Autodesk Fusion 360 part; units mm, degrees
(part 2 of 2)
  constraint coincident L500 L639.end
  constraint perpendicular L500 L639
  constraint coincident L499 L640.start
  constraint coincident L501 L640.end
  constraint perpendicular L501 L640
  constraint coincident L500 L641.end
  constraint perpendicular L500 L641
  constraint coincident L495 L642.end
  constraint perpendicular L495 L642
  constraint coincident L495 L643.end
  constraint perpendicular L495 L643
  constraint coincident L495 L644.start
  constraint coincident L496 L644.end
  constraint perpendicular L496 L644
  measures "d1" distance of L345 L502
  measures "d2" distance of L432 L500
  measures "d3" distance of L12 L501
  measures "d4" distance of L477 L499
  measures "d5" distance of L243 L498
  measures "d6" distance of L284 L497
  measures "d7" distance of L115 L496
  measures "d8" distance of L74 L495
  measures "d9" distance of L196 L494
  measures "d10" distance of L208 L493
extrude "Extrude1" add sketch "b27d7a26cd9df215f168af8e672502c9323f781d_switch" against normal blind 3 contours L51 L301 L303 L501 L579 | L40 L62 L499 L501 L580 L581 | L303 L500 L501 L630 | L301 L492 L499 L579 | L492 L498 L499 L635 | L303 L387 L500 L502 L620 | L32 L429 L499 L501 L582 L583 | L325 L492 L498 L635 | L303 L304 L320 L502 | L305 L325 L497 L635 | L373 L382 L500 L502 L618 L619 | L291 L302 L328 L498 L499 L634 | L436 L464 L499 L501 L584 L585 | L249 L497 L498 L578 L636 | L305 L323 L496 L497 | L320 L343 L500 L502 L605 | L347 L371 L500 L502 L616 L617 | L427 L484 L499 L501 L586 L587 | L141 L305 L495 L496 L528 | L256 L271 L497 L498 L576 L577 | L320 L500 L501 L641 | L305 L494 L495 L643 | L320 L356 L501 L640 | L342 L395 L500 L502 L606 L607 | L370 L417 L500 L502 L614 L615 | L485 L489 L499 L501 L588 L589 | L305 L493 L494 L637 | L98 L129 L495 L496 L529 L530 | L282 L314 L497 L498 L574 L575 | L356 L491 L499 L640 | L294 L305 L323 L493 | L291 L302 L328 L491 L498 L499 | L441 L499 L501 L604 L639 | L500 L501 L631 L639 | L385 L431 L500 L502 L608 L609 | L389 L413 L500 L502 L612 L613 | L358 L383 L388 L390 L398 L399 L400 L401 L405 L408 L409 L410 L411 L414 L416 L424 L425 L426 L428 L430 L500 L502 L611 L630 | L323 L494 L495 L642 | L178 L493 L494 L527 L638 | L80 L92 L495 L496 L531 L532 | L267 L281 L497 L498 L572 L573 | L293 L302 L307 L326 L337 L360 L491 L498 | L434 L458 L499 L590 L591 L633 | L377 L500 L502 L610 L631 | L54 L293 L302 L307 L323 L326 L337 L360 L497 L498 L555 | L443 L490 L499 L501 L602 L603 | L300 L334 L502 L628 L629 | L132 L323 L493 L494 L632 | L220 L221 L493 L494 L525 L526 | L64 L84 L495 L496 L533 L534 | L263 L318 L497 L498 L570 L571 | L467 L470 L499 L592 L593 L633 | L447 L468 L499 L600 L601 L633 | L354 L357 L502 L626 L627 | L358 L383 L388 L390 L398 L399 L400 L401 L405 L408 L410 L411 L414 L416 L424 L426 L428 L430 L611 | L287 L323 L495 L496 L554 | L9 L38 L497 L498 L556 L557 | L146 L156 L493 L494 L503 L504 | L215 L218 L493 L494 L523 L524 | L105 L125 L495 L496 L535 L536 | L236 L265 L497 L498 L568 L569 | L442 L474 L499 L594 L595 L633 | L462 L469 L499 L598 L599 L633 | L279 L313 L495 L496 L552 L553 | L56 L59 L497 L498 L558 L559 | L142 L187 L493 L494 L505 L506 | L206 L210 L493 L494 L521 L522 | L75 L107 L495 L496 L537 L538 | L273 L274 L497 L498 L566 L567 | L438 L463 L499 L596 L597 L633 | L261 L277 L495 L496 L550 L551 | L31 L37 L497 L498 L560 L561 | L124 L181 L493 L494 L507 L508 | L179 L217 L493 L494 L519 L520 | L96 L97 L495 L496 L539 L540 | L19 L280 L497 L498 L564 L565 | L230 L250 L495 L496 L548 L549 | L35 L258 L497 L498 L562 L563 | L184 L188 L493 L494 L509 L510 | L205 L213 L493 L494 L517 L518 | L116 L148 L495 L496 L541 L542 | L251 L253 L495 L496 L546 L547 | L191 L222 L493 L494 L511 L512 | L172 L174 L493 L494 L515 L516 | L68 L88 L495 L496 L543 L544 | L135 L240 L495 L496 L545 L644 | L211 L219 L493 L494 L513 L514 | L65 L69 L78 L86 L87 L91 L94 L103 L108 L117 L152 L163 L167 L170 L180 L182 L185 L186 L202 L212 | L67 L71 L76 L77 L83 L85 L90 L93 L99 L100 L101 L102 L104 L106 L109 L113 L118 L131 L149 L150 | L228 L229 L232 L239 L241 L242 L244 L246 L259 L264 L268 L269 L272 L275 L276 L285 L286 L290 L329 L330
extrude "Extrude2" add sketch "b27d7a26cd9df215f168af8e672502c9323f781d_switch" along normal blind 1.5 contours L5 L501 L579 L580 | L51 L301 L303 L501 L579 | L40 L62 L499 L501 L580 L581 | L58 L295 L297 L301 L316 L322 L499 L579 L580 | L303 L500 L501 L630 | L301 L492 L499 L579 | L295 L297 L301 L316 L322 L499 L579 | L295 L299 L308 L498 L499 L634 | L49 L501 L581 L582 | L492 L498 L499 L635 | L295 L299 L308 L498 L499 L635 | L303 L387 L500 L502 L620 | L452 L499 L581 L582 | L32 L429 L499 L501 L582 L583 | L325 L492 L498 L635 | L298 L299 L311 L312 L321 L325 L498 L635 | L303 L304 L320 L502 | L372 L500 L619 L620 | L406 L501 L583 L584 | L298 L299 L311 L312 L321 L325 L497 L498 L635 L636 | L305 L325 L497 L635 | L422 L502 L619 L620 | L373 L382 L500 L502 L618 L619 | L448 L499 L583 L584 | L291 L302 L328 L498 L499 L634 | L436 L464 L499 L501 L584 L585 | L249 L497 L498 L578 L636 | L305 L323 L496 L497 | L386 L500 L617 L618 | L42 L501 L585 L586 | L283 L498 L577 L578 | L320 L343 L500 L502 L605 | L412 L502 L617 L618 | L347 L371 L500 L502 L616 L617 | L488 L499 L585 L586 | L427 L484 L499 L501 L586 L587 | L141 L305 L495 L496 L528 | L256 L271 L497 L498 L576 L577 | L278 L497 L577 L578 | L320 L500 L501 L641 | L355 L502 L605 L606 | L420 L500 L615 L616 | L12 L501 L587 L588 | L305 L494 L495 L643 | L66 L496 L528 L529 | L237 L498 L575 L576 | L320 L356 L501 L640 | L500 L501 L639 L641 | L342 L395 L500 L502 L606 L607 | L359 L502 L615 L616 | L370 L417 L500 L502 L614 L615 | L477 L499 L587 L588 | L485 L489 L499 L501 L588 L589 | L305 L493 L494 L637 | L494 L495 L642 L643 | L98 L129 L495 L496 L529 L530 | L282 L314 L497 L498 L574 L575 | L296 L497 L575 L576 | L356 L491 L499 L640 | L291 L309 L317 L324 L356 L499 L501 L639 L640 | L341 L500 L605 L606 | L404 L502 L607 L608 | L348 L500 L613 L614 | L500 L501 L630 L631 | L451 L501 L589 L590 | L294 L305 L323 L493 | L493 L494 L637 L638 | L79 L495 L528 L529 | L112 L496 L530 L531 | L243 L498 L573 L574 | L291 L309 L317 L324 L356 L499 L640 | L291 L302 L328 L491 L498 L499 | L441 L499 L501 L604 L639 | L500 L501 L631 L639 | L385 L431 L500 L502 L608 L609 | L393 L502 L613 L614 | L389 L413 L500 L502 L612 L613 | L445 L499 L589 L590 | L501 L590 L591 L633 | L292 L306 L310 L315 L319 L327 L331 L332 L333 L334 L335 L336 L338 L339 L340 L346 L349 L350 L351 L352 L353 L354 L361 L362 L363 L364 L365 L366 L367 L368 L369 L500 L502 L624 L625 L626 L629 L630 L631 | L358 L383 L388 L390 L398 L399 L400 L401 L405 L408 L409 L410 L411 L414 L416 L424 L425 L426 L428 L430 L500 L502 L611 L630 | L323 L494 L495 L642 | L178 L493 L494 L527 L638 | L80 L92 L495 L496 L531 L532 | L267 L281 L497 L498 L572 L573 | L284 L497 L573 L574 | L293 L302 L307 L326 L337 L360 L491 L498 | L478 L501 L603 L604 | L394 L500 L607 L608 | L418 L502 L609 L610 | L432 L500 L611 L612 | L434 L458 L499 L590 L591 L633 | L471 L501 L591 L592 L633 | L377 L500 L502 L610 L631 | L226 L494 L526 L527 | L81 L495 L530 L531 | L95 L496 L532 L533 | L233 L498 L571 L572 | L54 L293 L302 L307 L323 L326 L337 L360 L497 L498 L555 | L443 L490 L499 L501 L602 L603 | L476 L499 L603 L604 | L345 L502 L611 L612 | L437 L499 L591 L592 | L501 L592 L593 L633 | L407 L500 L609 L610 | L501 L600 L601 L633 | L455 L501 L601 L602 | L300 L334 L502 L628 L629 | L132 L323 L493 L494 L632 | L203 L493 L526 L527 | L220 L221 L493 L494 L525 L526 | L64 L84 L495 L496 L533 L534 | L263 L318 L497 L498 L570 L571 | L231 L497 L571 L572 | L8 L498 L555 L556 | L467 L470 L499 L592 L593 L633 | L486 L501 L593 L594 L633 | L457 L501 L599 L600 L633 | L447 L468 L499 L600 L601 L633 | L354 L357 L502 L626 L627 | L358 L383 L388 L390 L398 L399 L400 L401 L405 L408 L410 L411 L414 L416 L424 L426 L428 L430 L611 | L344 L502 L627 L628 | L165 L493 L503 L632 | L173 L494 L524 L525 | L89 L495 L532 L533 | L70 L496 L534 L535 | L248 L498 L569 L570 | L287 L323 L495 L496 L554 | L17 L497 L555 L556 | L9 L38 L497 L498 L556 L557 | L454 L499 L601 L602 | L439 L499 L593 L594 | L501 L594 L595 L633 | L501 L598 L599 L633 | L160 L494 L503 L632 | L146 L156 L493 L494 L503 L504 | L209 L493 L524 L525 | L215 L218 L493 L494 L523 L524 | L105 L125 L495 L496 L535 L536 | L236 L265 L497 L498 L568 L569 | L247 L497 L569 L570 | L238 L496 L553 L554 | L53 L498 L557 L558 | L442 L474 L499 L594 L595 L633 | L453 L501 L595 L596 L633 | L483 L501 L597 L598 L633 | L462 L469 L499 L598 L599 L633 | L456 L499 L599 L600 | L289 L495 L553 L554 | L192 L493 L504 L505 | L196 L494 L522 L523 | L82 L495 L534 L535 | L115 L496 L536 L537 | L266 L498 L567 L568 | L279 L313 L495 L496 L552 L553 | L55 L497 L557 L558 | L56 L59 L497 L498 L558 L559 | L482 L499 L595 L596 | L501 L596 L597 L633 | L122 L494 L504 L505 | L142 L187 L493 L494 L505 L506 | L208 L493 L522 L523 | L206 L210 L493 L494 L521 L522 | L75 L107 L495 L496 L537 L538 | L273 L274 L497 L498 L566 L567 | L257 L497 L567 L568 | L288 L496 L551 L552 | L11 L498 L559 L560 | L438 L463 L499 L596 L597 L633 | L450 L499 L597 L598 | L260 L495 L551 L552 | L139 L493 L506 L507 | L175 L494 L520 L521 | L74 L495 L536 L537 | L73 L496 L538 L539 | L234 L498 L565 L566 | L261 L277 L495 L496 L550 L551 | L43 L497 L559 L560 | L31 L37 L497 L498 L560 L561 | L153 L494 L506 L507 | L124 L181 L493 L494 L507 L508 | L171 L493 L520 L521 | L179 L217 L493 L494 L519 L520 | L96 L97 L495 L496 L539 L540 | L19 L280 L497 L498 L564 L565 | L252 L497 L565 L566 | L270 L496 L549 L550 | L21 L498 L561 L562 | L227 L495 L549 L550 | L193 L493 L508 L509 | L224 L494 L518 L519 | L72 L495 L538 L539 | L154 L496 L540 L541 | L23 L498 L563 L564 | L230 L250 L495 L496 L548 L549 | L45 L497 L561 L562 | L35 L258 L497 L498 L562 L563 | L200 L494 L508 L509 | L184 L188 L493 L494 L509 L510 | L204 L493 L518 L519 | L205 L213 L493 L494 L517 L518 | L116 L148 L495 L496 L541 L542 | L44 L497 L563 L564 | L254 L496 L547 L548 | L262 L495 L547 L548 | L190 L493 L510 L511 | L183 L494 L516 L517 | L147 L495 L540 L541 | L138 L496 L542 L543 | L251 L253 L495 L496 L546 L547 | L223 L494 L510 L511 | L191 L222 L493 L494 L511 L512 | L225 L493 L516 L517 | L172 L174 L493 L494 L515 L516 | L68 L88 L495 L496 L543 L544 | L235 L496 L546 L644 | L255 L495 L546 L644 | L216 L493 L512 L513 | L197 L494 L514 L515 | L127 L495 L542 L543 | L111 L496 L544 L545 | L135 L240 L495 L496 L545 L644 | L189 L494 L512 L513 | L211 L219 L493 L494 L513 L514 | L214 L493 L514 L515 | L245 L495 L544 L545 | L65 L69 L78 L86 L87 L91 L94 L103 L108 L117 L152 L163 L167 L170 L180 L182 L185 L186 L202 L212 | L67 L71 L76 L77 L83 L85 L90 L93 L99 L100 L101 L102 L104 L106 L109 L113 L118 L131 L149 L150 | L228 L229 L232 L239 L241 L242 L244 L246 L259 L264 L268 L269 L272 L275 L276 L285 L286 L290 L329 L330
sketch "Sketch5" plane through (0, 0, 0) normal (0, 0, 1) x (1, 0, 0)
  line L0 (0.6891, 94.188) -> (284.6891, 94.188)
  line L1 (284.6891, 94.188) -> (284.6891, 1.188)
  line L2 (284.6891, 1.188) -> (0.6891, 1.188)
  line L3 (0.6891, 1.188) -> (0.6891, 94.188)
  dimension "d33" = 284
  dimension "d34" = 93
  constraint horizontal L0
  constraint vertical L1
  constraint horizontal L2
  constraint vertical L3
  measures "d33" distance of L0.start L0.end
  measures "d34" distance of L0.start L2.end
extrude "Extrude5" cut sketch "Sketch5" along normal blind -20 and the other way blind -20 keep common part
sketch "Sketch6" plane through (0, 0, -3) normal (0, 0, -1) x (1, 0, 0)
  line L0 (83.1067, -75.2429) -> (69.106, -75.2429)
  line L1 (69.106, -75.2429) -> (69.106, -58.2436)
  line L2 (69.106, -58.2436) -> (83.1067, -58.2436)
  line L3 (83.1067, -58.2436) -> (83.1067, -75.2429)
  line L4 (88.156, -75.2429) -> (88.156, -58.2436)
  line L5 (88.156, -58.2436) -> (102.157, -58.2436)
  line L6 (102.157, -58.2436) -> (102.157, -75.2429)
  line L7 (102.157, -75.2429) -> (88.156, -75.2429)
  line L8 (231.031, -37.1429) -> (231.031, -20.1435)
  line L9 (231.031, -20.1435) -> (245.032, -20.1435)
  line L10 (245.032, -20.1435) -> (245.032, -37.1429)
  line L11 (245.032, -37.1429) -> (250.081, -37.1429)
  line L12 (250.081, -37.1429) -> (250.081, -20.1435)
  line L13 (250.081, -20.1435) -> (264.08, -20.1435)
  line L14 (264.08, -20.1435) -> (264.08, -37.1429)
  line L15 (264.08, -37.1429) -> (269.131, -37.1429)
  line L16 (269.131, -37.1429) -> (269.131, -20.1435)
  line L17 (269.131, -20.1435) -> (283.13, -20.1435)
  line L18 (283.13, -20.1435) -> (283.13, -56.1929)
  line L19 (283.13, -56.1929) -> (245.032, -56.1929)
  line L20 (245.032, -56.1929) -> (245.032, -37.1429)
  line L21 (245.032, -37.1429) -> (231.031, -37.1429)
  line L22 (207.22, -56.1929) -> (207.22, -39.1922)
  line L23 (207.22, -39.1922) -> (221.219, -39.1922)
  line L24 (221.219, -39.1922) -> (221.219, -56.1929)
  line L25 (221.219, -56.1929) -> (207.22, -56.1929)
  line L26 (188.168, -56.1929) -> (188.168, -39.1922)
  line L27 (188.168, -39.1922) -> (202.168, -39.1922)
  line L28 (202.168, -39.1922) -> (202.168, -56.1929)
  line L29 (202.168, -56.1929) -> (188.168, -56.1929)
  line L30 (169.12, -56.1929) -> (169.12, -39.1922)
  line L31 (169.12, -39.1922) -> (183.119, -39.1922)
  line L32 (183.119, -39.1922) -> (183.119, -56.1929)
  line L33 (183.119, -56.1929) -> (169.12, -56.1929)
  line L34 (226.27, -56.1929) -> (226.27, -39.1922)
  line L35 (226.27, -39.1922) -> (240.269, -39.1922)
  line L36 (240.269, -39.1922) -> (240.269, -56.1929)
  line L37 (240.269, -56.1929) -> (226.27, -56.1929)
  line L38 (225.982, -37.1429) -> (211.981, -37.1429)
  line L39 (211.981, -37.1429) -> (211.981, -20.1435)
  line L40 (211.981, -20.1435) -> (225.982, -20.1435)
  line L41 (225.982, -20.1435) -> (225.982, -37.1429)
  line L42 (206.93, -37.1429) -> (192.931, -37.1429)
  line L43 (192.931, -37.1429) -> (192.931, -20.1435)
  line L44 (192.931, -20.1435) -> (206.93, -20.1435)
  line L45 (206.93, -20.1435) -> (206.93, -37.1429)
  line L46 (52.4372, -18.093) -> (52.4372, -1.5935)
  line L47 (52.4372, -1.5935) -> (66.4379, -1.5935)
  line L48 (66.4379, -1.5935) -> (66.4379, -18.093)
  line L49 (66.4379, -18.093) -> (52.4372, -18.093)
  line L50 (35.9538, -37.1429) -> (2.0385, -37.1429)
  line L51 (2.0385, -37.1429) -> (2.0385, -18.093)
  line L52 (2.0385, -18.093) -> (4.8121, -18.093)
  line L53 (4.8121, -18.093) -> (4.8121, -1.5935)
  line L54 (4.8121, -1.5935) -> (18.813, -1.5935)
  line L55 (18.813, -1.5935) -> (18.813, -18.093)
  line L56 (18.813, -18.093) -> (28.6246, -18.093)
  line L57 (28.6246, -18.093) -> (28.6246, -1.5935)
  line L58 (28.6246, -1.5935) -> (42.624, -1.5935)
  line L59 (42.624, -1.5935) -> (42.624, -18.093)
  line L60 (42.624, -18.093) -> (35.9538, -18.093)
  line L61 (35.9538, -18.093) -> (35.9538, -37.1429)
  line L62 (73.5803, -37.1429) -> (59.581, -37.1429)
  line L63 (59.581, -37.1429) -> (59.581, -20.1435)
  line L64 (59.581, -20.1435) -> (73.5803, -20.1435)
  line L65 (73.5803, -20.1435) -> (73.5803, -1.5935)
  line L66 (73.5803, -1.5935) -> (85.3237, -1.5935)
  line L67 (85.3237, -1.5935) -> (85.3237, -7.2775)
  line L68 (85.3237, -7.2775) -> (123.91, -7.2775)
  line L69 (123.91, -7.2775) -> (123.91, -1.5935)
  line L70 (123.91, -1.5935) -> (137.909, -1.5935)
  line L71 (137.909, -1.5935) -> (137.909, -7.2775)
  line L72 (137.909, -7.2775) -> (176.5478, -7.2775)
  line L73 (176.5478, -7.2775) -> (176.5478, -1.5935)
  line L74 (176.5478, -1.5935) -> (187.882, -1.5935)
  line L75 (187.882, -1.5935) -> (187.882, -37.1429)
  line L76 (187.882, -37.1429) -> (173.881, -37.1429)
  line L77 (173.881, -37.1429) -> (173.881, -21.6435)
  line L78 (173.881, -21.6435) -> (168.83, -21.6435)
  line L79 (168.83, -21.6435) -> (168.83, -37.1429)
  line L80 (168.83, -37.1429) -> (154.831, -37.1429)
  line L81 (154.831, -37.1429) -> (154.831, -21.6435)
  line L82 (154.831, -21.6435) -> (149.782, -21.6435)
  line L83 (149.782, -21.6435) -> (149.782, -37.1429)
  line L84 (149.782, -37.1429) -> (135.781, -37.1429)
  line L85 (135.781, -37.1429) -> (135.781, -21.6435)
  line L86 (135.781, -21.6435) -> (130.732, -21.6435)
  line L87 (130.732, -21.6435) -> (130.732, -37.1429)
  line L88 (130.732, -37.1429) -> (116.731, -37.1429)
  line L89 (116.731, -37.1429) -> (116.731, -21.6435)
  line L90 (116.731, -21.6435) -> (111.682, -21.6435)
  line L91 (111.682, -21.6435) -> (111.682, -37.1429)
  line L92 (111.682, -37.1429) -> (97.681, -37.1429)
  line L93 (97.681, -37.1429) -> (97.681, -21.6435)
  line L94 (97.681, -21.6435) -> (92.6317, -21.6435)
  line L95 (92.6317, -21.6435) -> (92.6317, -37.1429)
  line L96 (92.6317, -37.1429) -> (78.631, -37.1429)
  line L97 (78.631, -37.1429) -> (78.631, -21.6435)
  line L98 (78.631, -21.6435) -> (73.5803, -21.6435)
  line L99 (73.5803, -21.6435) -> (73.5803, -37.1429)
  line L100 (192.931, -18.093) -> (192.931, -1.5935)
  line L101 (192.931, -1.5935) -> (206.93, -1.5935)
  line L102 (206.93, -1.5935) -> (206.93, -18.093)
  line L103 (206.93, -18.093) -> (192.931, -18.093)
  line L104 (211.981, -18.093) -> (211.981, -1.5935)
  line L105 (211.981, -1.5935) -> (225.982, -1.5935)
  line L106 (225.982, -1.5935) -> (225.982, -18.093)
  line L107 (225.982, -18.093) -> (211.981, -18.093)
  line L108 (231.031, -18.093) -> (231.031, -1.5935)
  line L109 (231.031, -1.5935) -> (245.032, -1.5935)
  line L110 (245.032, -1.5935) -> (245.032, -18.093)
  line L111 (245.032, -18.093) -> (231.031, -18.093)
  line L112 (250.081, -18.093) -> (250.081, -1.5935)
  line L113 (250.081, -1.5935) -> (264.08, -1.5935)
  line L114 (264.08, -1.5935) -> (264.08, -18.093)
  line L115 (264.08, -18.093) -> (250.081, -18.093)
  line L116 (54.5317, -37.1429) -> (40.531, -37.1429)
  line L117 (40.531, -37.1429) -> (40.531, -20.1435)
  line L118 (40.531, -20.1435) -> (54.5317, -20.1435)
  line L119 (54.5317, -20.1435) -> (54.5317, -37.1429)
  line L120 (269.131, -18.093) -> (269.131, -1.5935)
  line L121 (269.131, -1.5935) -> (283.13, -1.5935)
  line L122 (283.13, -1.5935) -> (283.13, -18.093)
  line L123 (283.13, -18.093) -> (269.131, -18.093)
  line L124 (9.576, -56.1929) -> (9.576, -39.1922)
  line L125 (9.576, -39.1922) -> (23.5755, -39.1922)
  line L126 (23.5755, -39.1922) -> (23.5755, -56.1929)
  line L127 (23.5755, -56.1929) -> (9.576, -56.1929)
  line L128 (35.7699, -56.1929) -> (35.7699, -39.1922)
  line L129 (35.7699, -39.1922) -> (49.7692, -39.1922)
  line L130 (49.7692, -39.1922) -> (49.7692, -56.1929)
  line L131 (49.7692, -56.1929) -> (35.7699, -56.1929)
  line L132 (54.8171, -56.1929) -> (54.8171, -39.1922)
  line L133 (54.8171, -39.1922) -> (68.8178, -39.1922)
  line L134 (68.8178, -39.1922) -> (68.8178, -56.1929)
  line L135 (68.8178, -56.1929) -> (54.8171, -56.1929)
  line L136 (73.8685, -56.1929) -> (73.8685, -39.1922)
  line L137 (73.8685, -39.1922) -> (87.8678, -39.1922)
  line L138 (87.8678, -39.1922) -> (87.8678, -56.1929)
  line L139 (87.8678, -56.1929) -> (73.8685, -56.1929)
  line L140 (131.018, -56.1929) -> (131.018, -39.1922)
  line L141 (131.018, -39.1922) -> (145.018, -39.1922)
  line L142 (145.018, -39.1922) -> (145.018, -56.1929)
  line L143 (145.018, -56.1929) -> (131.018, -56.1929)
  line L144 (150.068, -56.1929) -> (150.068, -39.1922)
  line L145 (150.068, -39.1922) -> (164.068, -39.1922)
  line L146 (164.068, -39.1922) -> (164.068, -56.1929)
  line L147 (164.068, -56.1929) -> (150.068, -56.1929)
  line L148 (111.967, -56.1929) -> (111.967, -39.1922)
  line L149 (111.967, -39.1922) -> (125.969, -39.1922)
  line L150 (125.969, -39.1922) -> (125.969, -56.1929)
  line L151 (125.969, -56.1929) -> (111.967, -56.1929)
  line L152 (92.9185, -56.1929) -> (92.9185, -39.1922)
  line L153 (92.9185, -39.1922) -> (106.918, -39.1922)
  line L154 (106.918, -39.1922) -> (106.918, -56.1929)
  line L155 (106.918, -56.1929) -> (92.9185, -56.1929)
  line L156 (16.4317, -93.7929) -> (2.4309, -93.7929)
  line L157 (2.4309, -93.7929) -> (2.4309, -77.2936)
  line L158 (2.4309, -77.2936) -> (16.4317, -77.2936)
  line L159 (16.4317, -77.2936) -> (16.4317, -93.7929)
  line L160 (116.731, -93.7929) -> (116.731, -77.2936)
  line L161 (116.731, -77.2936) -> (130.732, -77.2936)
  line L162 (130.732, -77.2936) -> (130.732, -93.7929)
  line L163 (130.732, -93.7929) -> (116.731, -93.7929)
  line L164 (154.831, -93.7929) -> (154.831, -77.2936)
  line L165 (154.831, -77.2936) -> (168.83, -77.2936)
  line L166 (168.83, -77.2936) -> (168.83, -93.7929)
  line L167 (168.83, -93.7929) -> (154.831, -93.7929)
  line L168 (21.4809, -93.7929) -> (21.4809, -77.2936)
  line L169 (21.4809, -77.2936) -> (35.4817, -77.2936)
  line L170 (35.4817, -77.2936) -> (35.4817, -93.7929)
  line L171 (35.4817, -93.7929) -> (21.4809, -93.7929)
  line L172 (192.931, -93.7929) -> (192.931, -77.2936)
  line L173 (192.931, -77.2936) -> (206.93, -77.2936)
  line L174 (206.93, -77.2936) -> (206.93, -93.7929)
  line L175 (206.93, -93.7929) -> (192.931, -93.7929)
  line L176 (97.681, -93.7929) -> (97.681, -77.2936)
  line L177 (97.681, -77.2936) -> (111.682, -77.2936)
  line L178 (111.682, -77.2936) -> (111.682, -93.7929)
  line L179 (111.682, -93.7929) -> (97.681, -93.7929)
  line L180 (173.881, -93.7929) -> (173.881, -77.2936)
  line L181 (173.881, -77.2936) -> (187.882, -77.2936)
  line L182 (187.882, -77.2936) -> (187.882, -93.7929)
  line L183 (187.882, -93.7929) -> (173.881, -93.7929)
  line L184 (59.581, -93.7929) -> (59.581, -77.2936)
  line L185 (59.581, -77.2936) -> (73.5803, -77.2936)
  line L186 (73.5803, -77.2936) -> (73.5803, -93.7929)
  line L187 (73.5803, -93.7929) -> (59.581, -93.7929)
  line L188 (78.631, -93.7929) -> (78.631, -77.2936)
  line L189 (78.631, -77.2936) -> (92.6317, -77.2936)
  line L190 (92.6317, -77.2936) -> (92.6317, -93.7929)
  line L191 (92.6317, -93.7929) -> (78.631, -93.7929)
  line L192 (40.531, -93.7929) -> (40.531, -77.2936)
  line L193 (40.531, -77.2936) -> (54.5317, -77.2936)
  line L194 (54.5317, -77.2936) -> (54.5317, -93.7929)
  line L195 (54.5317, -93.7929) -> (40.531, -93.7929)
  line L196 (211.981, -93.7929) -> (211.981, -77.2936)
  line L197 (211.981, -77.2936) -> (225.982, -77.2936)
  line L198 (225.982, -77.2936) -> (225.982, -93.7929)
  line L199 (225.982, -93.7929) -> (211.981, -93.7929)
  line L200 (135.781, -93.7929) -> (135.781, -77.2936)
  line L201 (135.781, -77.2936) -> (149.782, -77.2936)
  line L202 (149.782, -77.2936) -> (149.782, -93.7929)
  line L203 (149.782, -93.7929) -> (135.781, -93.7929)
  line L204 (178.357, -75.2429) -> (164.356, -75.2429)
  line L205 (164.356, -75.2429) -> (164.356, -58.2436)
  line L206 (164.356, -58.2436) -> (178.357, -58.2436)
  line L207 (178.357, -58.2436) -> (178.357, -75.2429)
  line L208 (64.0567, -75.2429) -> (50.056, -75.2429)
  line L209 (50.056, -75.2429) -> (50.056, -58.2436)
  line L210 (50.056, -58.2436) -> (64.0567, -58.2436)
  line L211 (64.0567, -58.2436) -> (64.0567, -75.2429)
  line L212 (121.205, -75.2429) -> (107.206, -75.2429)
  line L213 (107.206, -75.2429) -> (107.206, -58.2436)
  line L214 (107.206, -58.2436) -> (121.205, -58.2436)
  line L215 (121.205, -58.2436) -> (121.205, -75.2429)
  line L216 (140.257, -75.2429) -> (126.256, -75.2429)
  line L217 (126.256, -75.2429) -> (126.256, -58.2436)
  line L218 (126.256, -58.2436) -> (140.257, -58.2436)
  line L219 (140.257, -58.2436) -> (140.257, -75.2429)
  line L220 (21.1942, -75.2429) -> (7.1947, -75.2429)
  line L221 (7.1947, -75.2429) -> (7.1947, -58.2436)
  line L222 (7.1947, -58.2436) -> (21.1942, -58.2436)
  line L223 (21.1942, -58.2436) -> (21.1942, -75.2429)
  line L224 (159.305, -75.2429) -> (145.306, -75.2429)
  line L225 (145.306, -75.2429) -> (145.306, -58.2436)
  line L226 (145.306, -58.2436) -> (159.305, -58.2436)
  line L227 (159.305, -58.2436) -> (159.305, -75.2429)
  line L228 (45.0053, -75.2429) -> (31.0059, -75.2429)
  line L229 (31.0059, -75.2429) -> (31.0059, -58.2436)
  line L230 (31.0059, -58.2436) -> (45.0053, -58.2436)
  line L231 (45.0053, -58.2436) -> (45.0053, -75.2429)
  line L232 (235.507, -75.2429) -> (221.506, -75.2429)
  line L233 (221.506, -75.2429) -> (221.506, -58.2436)
  line L234 (221.506, -58.2436) -> (235.507, -58.2436)
  line L235 (235.507, -58.2436) -> (235.507, -75.2429)
  line L236 (231.031, -93.7929) -> (231.031, -77.2936)
  line L237 (231.031, -77.2936) -> (245.032, -77.2936)
  line L238 (245.032, -77.2936) -> (245.032, -93.7929)
  line L239 (245.032, -93.7929) -> (231.031, -93.7929)
  line L240 (216.455, -75.2429) -> (202.456, -75.2429)
  line L241 (202.456, -75.2429) -> (202.456, -58.2436)
  line L242 (202.456, -58.2436) -> (216.455, -58.2436)
  line L243 (216.455, -58.2436) -> (216.455, -75.2429)
  line L244 (197.407, -75.2429) -> (183.406, -75.2429)
  line L245 (183.406, -75.2429) -> (183.406, -58.2436)
  line L246 (183.406, -58.2436) -> (197.407, -58.2436)
  line L247 (197.407, -58.2436) -> (197.407, -75.2429)
  line L248 (249, -93.7929) -> (249, -75.2429)
  line L249 (249, -75.2429) -> (240.556, -75.2429)
  line L250 (240.556, -75.2429) -> (240.556, -58.2436)
  line L251 (240.556, -58.2436) -> (254.555, -58.2436)
  line L252 (254.555, -58.2436) -> (254.555, -75.2429)
  line L253 (254.555, -75.2429) -> (264.368, -75.2429)
  line L254 (264.368, -75.2429) -> (264.368, -58.2436)
  line L255 (264.368, -58.2436) -> (278.368, -58.2436)
  line L256 (278.368, -58.2436) -> (278.368, -75.2429)
  line L257 (278.368, -75.2429) -> (283.13, -75.2429)
  line L258 (283.13, -75.2429) -> (283.13, -93.7929)
  line L259 (283.13, -93.7929) -> (249, -93.7929)
  line L260 (284.6891, -94.188) -> (284.6891, -1.188)
  line L261 (284.6891, -1.188) -> (0.6891, -1.188)
  line L262 (0.6891, -1.188) -> (0.6891, -94.188)
  line L263 (0.6891, -94.188) -> (284.6891, -94.188)
  line L264 (190.3711, 5.0161) -> (190.3711, -38.1596)
  line L265 (190.3711, -38.1596) -> (147.5827, -38.1596)
  line L266 (147.5827, -38.1596) -> (147.5827, -57.2129)
  line L267 (147.5827, -57.2129) -> (180.9987, -57.2129)
  line L268 (180.9987, -57.2129) -> (180.8812, -76.2514)
  line L269 (180.8812, -76.2514) -> (152.2181, -76.2514)
  line L270 (152.2181, -76.2514) -> (152.2181, -102)
  line L271 (152.2181, -102) -> (301.844, -102)
  line L272 (301.844, -102) -> (305, 10)
  line L273 (305, 10) -> (190.3711, 5.0161)
  constraint perpendicular L261 L264
  constraint perpendicular L83 L265
  constraint perpendicular L226 L266
  constraint perpendicular L266 L267
  constraint perpendicular L162 L269
  constraint perpendicular L263 L270
  constraint perpendicular L198 L271
named bodies: "Plate"
